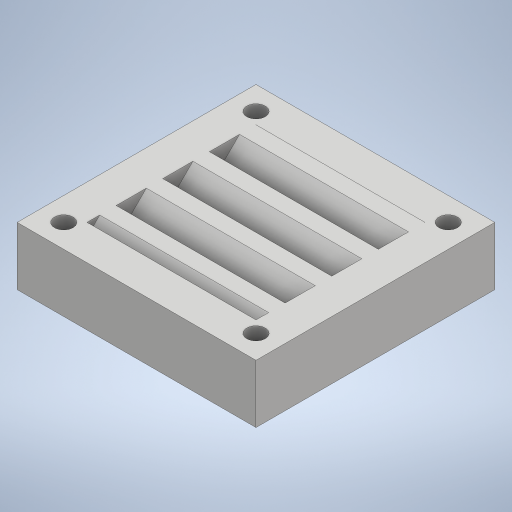
# Autodesk Inventor part: Trampa de luz
Saved by Autodesk Inventor 2024.2 (Build 282272000, 272)
## iProperties
Created: 2025-09-19
Part Number: Trampa de luz
Material: Genérico
Document SubType Name: Modeling
Designer: jd.castellanosq
Density: 1 g/cm^3
Appearance: Valor por defecto
Author: jd.castellanosq
Autodesk Inventor part; units mm, degrees
ref_plane "YZ Plane" through (0, 0, 0) normal (1, 0, 0) x (0, 1, 0)
ref_plane "XZ Plane" through (0, 0, 0) normal (0, 1, 0) x (-1, 0, 0)
ref_plane "XY Plane" through (0, 0, 0) normal (0, 0, 1) x (1, 0, 0)
sketch "Boceto3" plane through (0, 0, 0) normal (0, 0, 1) x (1, 0, 0)
  line L0 (-20.5, 20.5) -> (20.5, 20.5)
  line L1 (20.5, 20.5) -> (20.5, -20.5)
  line L2 (20.5, -20.5) -> (-20.5, -20.5)
  line L3 (-20.5, -20.5) -> (-20.5, 20.5)
  line L4 (14.5, 14.5) -> (-14.5, 14.5)
  line L5 (-14.5, 14.5) -> (-14.5, -14.5)
  line L6 (-14.5, -14.5) -> (14.5, -14.5)
  line L7 (14.5, -14.5) -> (14.5, 14.5)
  circle A0 centre (-16.5, 16.5) radius 1.6
  circle A1 centre (16.5, 16.5) radius 1.6
  circle A2 centre (-16.5, -16.5) radius 1.6
  circle A3 centre (16.5, -16.5) radius 1.6
  point P0 (0, 0)
  point P1 (0, 20.5)
  point P2 (20.5, 0)
  dimension "d22" = 41
  dimension "d23" = 6
  dimension "d25" = 3.2
  dimension "d31" = 33
  dimension "d32" = 16.5
  dimension "d33" = 16.5
  dimension "d34" = 33
  constraints: 16 end point, 4 centre point, 4 parallel, 3 equal radius, 3 horizontal alignment, 3 perpendicular, 3 vertical alignment, 2 midpoint, 1 horizontal, 3 other
  measures "d22" distance of L2.end L0.start
  measures "d23" distance between parallel lines of L0 L4
  measures "d25" diameter of A0
  measures "d31" distance of A1.centre A0.centre
  measures "d32" horizontal distance of point (0, 0) A1.centre
  measures "d33" horizontal distance of A0.centre point (0, 0)
  measures "d34" distance of A0.centre A2.centre
extrude "Extrusión3" add sketch "Boceto3" along normal blind 10
sketch "Boceto4" plane through (-14.5, -14.5, 0) normal (1, 0, 0) x (0, 0, -1)
  line L0 (0, 0) -> (-10, 0) projected
  line L1 (-10, 0) -> (-10, 29) projected
  line L2 (0, 29) -> (-10, 29) projected
  line L3 (0, 0) -> (0, 29) projected
  line L4 (-10, 29) -> (-5, 24)
  line L5 (-5, 24) -> (0, 29)
  line L6 (-10, 26.1716) -> (-5, 21.1716)
  line L7 (-5, 21.1716) -> (0, 26.1716)
  line L8 (-10, 26.1716) -> (-10, 29)
  line L9 (-10, 35) -> (-10, -6) projected
  line L10 (0, 26.1716) -> (0, 29)
  line L11 (0, 35) -> (0, -6) projected
  line L12 (-10, 18.1716) -> (-10, 21)
  line L13 (-10, 21) -> (-5, 16)
  line L14 (-10, 18.1716) -> (-5, 13.1716)
  line L15 (-5, 13.1716) -> (0, 18.1716)
  line L16 (-5, 16) -> (0, 21)
  line L17 (0, 18.1716) -> (0, 21)
  line L18 (-10, 10.1716) -> (-10, 13)
  line L19 (-10, 13) -> (-5, 8)
  line L20 (-10, 10.1716) -> (-5, 5.1716)
  line L21 (-5, 5.1716) -> (0, 10.1716)
  line L22 (-5, 8) -> (0, 13)
  line L23 (0, 10.1716) -> (0, 13)
  line L24 (-10, 2.1716) -> (-10, 5)
  line L25 (-10, 5) -> (-5, 0)
  line L26 (-10, 2.1716) -> (-5, -2.8284)
  line L27 (-5, -2.8284) -> (0, 2.1716)
  line L28 (-5, 0) -> (0, 5)
  line L29 (0, 2.1716) -> (0, 5)
  point P0 (0, 14.5)
  point P1 (-5, 29)
  point P2 (0, 10.1716)
  point P3 (0, 18.1716)
  dimension "d39" = 2
  dimension "d42" = 8
  constraints: 48 end point, 2 collinear, 2 perpendicular, 2 point on line, 2 vertical alignment, 1 midpoint, 1 vertical, 36 other
  measures "d39" distance between parallel lines of L4 L6
  measures "d42" distance of L6.start L12.start
extrude "Extrusión4" add sketch "Boceto4" along normal up to surface (29 mm away) contours L27 L26 L0 | L0 L28 L3 L27 | L0 L26 L1 L25 | L21 L20 L1 L19 L22 L3 | L15 L14 L1 L13 L16 L3 | L7 L6 L1 L4 L5 L3
equation "\"d32\" = 0.5 * d31"
equation "\"d33\" = d32"
equation "\"d34\" = d31"
